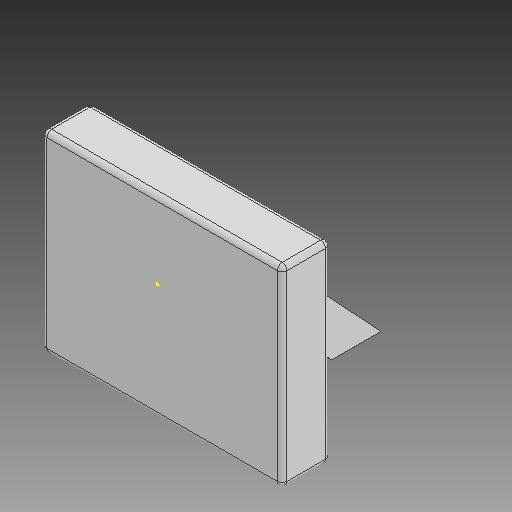
# Autodesk Inventor part: Lampe
Saved by Autodesk Inventor 2021 (Build 250183000, 183)
## iProperties
Created: 2022-03-14
Part Number: Lampe
Material: Generisch
Document SubType Name: Modeling
Designer: lukas
Density: 1 g/cm^3
Appearance: Vorgabe
Stock Number: Licht
Author: lukas
Autodesk Inventor part; units mm, degrees
ref_plane "XZ Plane" through (0, 0, 0) normal (0, 1, 0) x (-1, 0, 0)
ref_plane "XY Plane" through (0, 0, 0) normal (0, 0, 1) x (1, 0, 0)
sketch "Skizze1" plane through (0, 0, 0) normal (0, 0, 1) x (1, 0, 0)
  line L0 (-68.1013, 0) -> (71.8987, 0) projected
  line L1 (0, -64.8603) -> (0, 47.8406) projected
  line L2 (-48.1013, 31.7405) -> (51.8987, 31.7405)
  line L3 (51.8987, 31.7405) -> (51.8987, -48.2595)
  line L4 (51.8987, -48.2595) -> (-48.1013, -48.2595)
  line L5 (-48.1013, -48.2595) -> (-48.1013, 31.7405)
  point P0 (0, 0)
  dimension "d0" = 100
  dimension "d1" = 80
  constraints: 8 end point, 2 parallel, 1 horizontal, 1 perpendicular
  measures "d0" distance between parallel lines of L3 L5
  measures "d1" distance between parallel lines of L2 L4
extrude "Extrusion1" add sketch "Skizze1" along normal blind 20
fillet "Rundung1" radius 2 4 edges at (1.8987, 31.7405, 20) (-48.1013, -8.2595, 20) (51.8987, -8.2595, 20) (1.8987, -48.2595, 20)
fillet "Rundung2" radius 2 12 edges at (51.8987, -8.2595, 0) (1.8987, 31.7405, 0) (1.8987, -48.2595, 0) (-48.1013, -8.2595, 0) (51.3129, 31.1547, 19.4142) (51.8987, 31.7405, 9) (-47.5155, 31.1547, 19.4142) (-48.1013, 31.7405, 9) (51.3129, -47.6737, 19.4142) (51.8987, -48.2595, 9) (-47.5155, -47.6737, 19.4142) (-48.1013, -48.2595, 9)
sketch "Skizze2" plane through (0, 0, 0) normal (0, 0, -1) x (-1, 0, 0)
  line L0 (16.1013, 1.7405) -> (16.1013, -18.2595)
  line L1 (-19.8987, -18.2595) -> (-19.8987, 1.7405)
  line L2 (-49.8987, 29.7405) -> (46.1013, 29.7405) projected
  line L3 (-49.8987, -46.2595) -> (-49.8987, 29.7405) projected
  line L4 (46.1013, 29.7405) -> (46.1013, -46.2595) projected
  line L5 (-14.8987, -18.2595) -> (-14.8987, 1.7405)
  line L6 (11.1013, -18.2595) -> (11.1013, 1.7405)
  line L7 (-19.8987, 1.7405) -> (-14.8987, 1.7405)
  line L8 (11.1013, 1.7405) -> (16.1013, 1.7405)
  line L9 (16.1013, -18.2595) -> (11.1013, -18.2595)
  line L10 (-14.8987, -18.2595) -> (-19.8987, -18.2595)
  point P0 (0, 0)
  dimension "d8" = 30
  dimension "d9" = 30
  dimension "d10" = 5
  dimension "d11" = 5
  dimension "d12" = 20
  dimension "d13" = 20
  constraints: 16 end point, 6 perpendicular, 5 parallel, 2 horizontal
  measures "d8" distance between parallel lines of L1 L3
  measures "d9" distance between parallel lines of L4 L0
  measures "d10" distance between parallel lines of L5 L1
  measures "d11" distance between parallel lines of L0 L6
  measures "d12" distance between parallel lines of L7 L10
  measures "d13" distance between parallel lines of L8 L9
extrude "Extrusion2" add sketch "Skizze2" along normal blind 20
fillet "Rundung3" radius 5 4 edges at (17.3987, 1.7405, -20) (17.3987, -18.2595, -20) (-13.6013, 1.7405, -20) (-13.6013, -18.2595, -20)
sketch "Skizze3" plane through (0, 0, 20) normal (0, 0, 1) x (1, 0, 0)
  point P0 (0, 0)
sketch "Skizze4" plane through (19.8987, -18.2595, 0) normal (1, 0, 0) x (0, 0, -1)
  line L0 (0, 0) -> (15, 0) projected
  line L1 (20, 15) -> (20, 5) projected
  circle A0 centre (10, 10) radius 2.5
  point P0 (0, 18.2595)
  dimension "d17" = 10
  dimension "d18" = 10
  dimension "d19" = 5
  constraints: 1 centre point, 1 coincident
  measures "d17" distance from line of point (10, 10) L0
  measures "d18" distance from line of point (10, 10) L1
  measures "d19" diameter of A0
extrude "Extrusion3" cut sketch "Skizze4" against normal blind 40
sketch "Skizze5" plane through (19.8987, -18.2595, 0) normal (1, 0, 0) x (0, 0, -1)
  point P0 (0, 18.2595)
ref_plane "Arbeitsebene1" through (14.88, 0, 0) normal (1, 0, 0) x (0, 1, 0)
sketch "Skizze6" plane through (14.88, 0, 0) normal (1, 0, 0) x (0, 1, 0)
  line L0 (-7.91, 0.6008) -> (-48.7601, -37.6418)
  line L1 (-48.7601, -58.1892) -> (2.3413, -10.3495)
  line L2 (2.3413, -10.3495) -> (-7.91, 0.6008)
  circle A0 centre (-8.2595, -10) radius 2.5 projected
  line L3 (-48.7601, -58.1892) -> (-48.7601, -37.6418)
  point P0 (0, 0)
  dimension "d23" = 7.5
  dimension "d24" = 7.5
  dimension "d25" = 15
  dimension "d26" = 70
  dimension "d27" = 46.888
  constraints: 9 end point, 1 perpendicular, 1 vertical
  measures "d23" distance from line of L2 A0.centre
  measures "d24" distance from line of A0.centre L0
  measures "d25" distance between parallel lines of L1 L0
  measures "d26" distance from line of L1.start L2
  measures "d27" angle of L1 L3
extrude "Extrusion4" add sketch "Skizze6" against normal blind 25.98 contours L2 L1 L3 L0 | A0
fillet "Rundung4" radius 5 1 edges at (1.89, 2.3413, -10.3495)
sketch "Skizze7" plane through (-11.1, 0, 0) normal (-1, 0, 0) x (0, 0, 1)
  circle A0 centre (-10, -8.2595) radius 2.5 projected
  circle A1 centre (-10, -8.2595) radius 2.5
  point P0 (0, 0)
  point P1 (-10.0246, -8.2595)
  dimension "d31" = 0
  constraints: 1 centre point, 1 coincident, 1 concentric
  measures "d31" vertical distance of point (-10.025, -8.259) A0.centre
extrude "Extrusion5" add sketch "Skizze7" along normal blind 5
sketch "Skizze8" plane through (14.88, 0, 0) normal (1, 0, 0) x (0, 0, -1)
  circle A0 centre (10, -8.2595) radius 2.5 projected
  circle A1 centre (10, -8.2595) radius 2.5
  point P0 (0, 0)
  point P1 (9.9522, -8.2595)
  dimension "d34" = 0
  constraints: 1 centre point, 1 coincident
  measures "d34" vertical distance of A0.centre point (9.952, -8.259)
extrude "Extrusion6" add sketch "Skizze8" along normal blind 5
